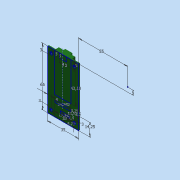
# Autodesk Inventor part: Motherboard_dummy
Saved by Autodesk Inventor 2015 (Build 190159000, 159)
## iProperties
Created: 2014-12-25
Part Number: Motherboard_dummy
Material: ABS Plastic
Document SubType Name: Modeling
Designer: Openlab
Density: 1.06 g/cm^3
Appearance: Smooth - Dark Forest Green
Author: Openlab
Autodesk Inventor part; units mm, degrees
ref_plane "YZ Plane" through (0, 0, 0) normal (1, 0, 0) x (0, 1, 0)
ref_plane "XZ Plane" through (0, 0, 0) normal (0, 1, 0) x (-1, 0, 0)
ref_plane "XY Plane" through (0, 0, 0) normal (0, 0, 1) x (1, 0, 0)
sketch "Sketch1" plane through (0, 0, 0) normal (0, 1, 0) x (-1, 0, 0)
  line L0 (0, 0) -> (0, -65)
  line L1 (35, -65) -> (35, 0)
  line L2 (35, 0) -> (0, 0)
  line L3 (0, -65) -> (35, -65)
  line L4 (27.271, 0) -> (8.729, 0)
  line L5 (8.729, 0) -> (8.729, -43.18)
  line L6 (8.729, -43.18) -> (27.271, -43.18)
  line L7 (27.271, -43.18) -> (27.271, 0)
  line L8 (18, 6.7089) -> (18, -52.768) construction
  line L9 (22, -5) -> (14, -5)
  line L10 (14, -5) -> (14, 0)
  line L11 (14, 0) -> (22, 0)
  line L12 (22, 0) -> (22, -5)
  circle A0 centre (31, -60) radius 1.5
  circle A1 centre (5, -60) radius 1.5
  circle A2 centre (31, -5) radius 1.5
  circle A3 centre (5, -5) radius 1.5
  line L13 (26.75, -48.25) -> (9.25, -48.25)
  line L14 (9.25, -48.25) -> (9.25, -50.75)
  line L15 (9.25, -50.75) -> (26.75, -50.75)
  line L16 (26.75, -50.75) -> (26.75, -48.25)
  line L17 (20.85, -55.75) -> (10.85, -55.75)
  line L18 (10.85, -55.75) -> (10.85, -58.25)
  line L19 (10.85, -58.25) -> (20.85, -58.25)
  line L20 (20.85, -58.25) -> (20.85, -55.75)
  point P0 (-55, 5)
  dimension "d0" = 35
  dimension "d1" = 65
  dimension "d2" = 5
  dimension "d3" = 4
  dimension "d4" = 5
  dimension "d5" = 5
  dimension "d6" = 18.542
  dimension "d7" = 43.18
  dimension "d8" = 8
  dimension "d9" = 5
  dimension "d10" = 55
  dimension "d11" = 5
  dimension "d12" = 18
  dimension "d13" = 3
  dimension "d14" = 3
  dimension "d15" = 3
  dimension "d16" = 3
  dimension "d23" = 17.5
  dimension "d24" = 2.5
  dimension "d25" = 9.25
  dimension "d26" = 14.25
  dimension "d27" = 10
  dimension "d28" = 2.5
  dimension "d29" = 10.85
  dimension "d30" = 6.75
  constraints: 42 end point, 10 parallel, 6 coincident, 5 horizontal, 5 perpendicular, 4 centre point, 4 horizontal alignment, 2 vertical alignment, 1 vertical, 2 other
  measures "d0" distance of L1.start L0.end
  measures "d1" distance of L1.end L1.start
  measures "d2" distance from line of L2 point (31, -5)
  measures "d3" distance from line of L1 point (31, -60)
  measures "d4" distance from line of L3 point (31, -60)
  measures "d5" distance from line of L0 point (5, -5)
  measures "d6" distance of L5.end L6.end
  measures "d7" distance of L4.end L5.end
  measures "d8" distance of L9.start L9.end
  measures "d9" distance of L11.end L9.start
  measures "d10" distance from line of point (-55, 5) L0
  measures "d11" vertical distance of point (-55, 5) point (0, 0)
  measures "d12" distance between parallel lines of L8 L0
  measures "d13" diameter of A0
  measures "d14" diameter of A1
  measures "d15" diameter of A2
  measures "d16" diameter of A3
  measures "d23" distance of L15.end L14.end
  measures "d24" distance of L14.end L13.end
  measures "d25" distance between parallel lines of L0 L14
  measures "d26" distance between parallel lines of L3 L15
  measures "d27" distance of L19.end L18.end
  measures "d28" distance of L18.end L17.end
  measures "d29" distance between parallel lines of L0 L18
  measures "d30" distance between parallel lines of L3 L19
extrude "Extrusion1" add sketch "Sketch1" along normal blind 1.5 contours L2 L5 L6 L7 L1 L3 L0 | L2 L10 L9 L12 L7 L6 L5 | L2 L12 L9 L10 | L16 L15 L14 L13 | L20 L19 L18 L17
extrude "Extrusion2" add sketch "Sketch1" along normal blind 5 contours L2 L10 L9 L12 L7 L6 L5 | L2 L12 L9 L10
extrude "Extrusion3" add sketch "Sketch1" along normal blind 7 contours L2 L12 L9 L10
extrude "Extrusion4" add sketch "Sketch1" along normal blind 10 contours L16 L15 L14 L13 | L20 L19 L18 L17
body "Solid1"
